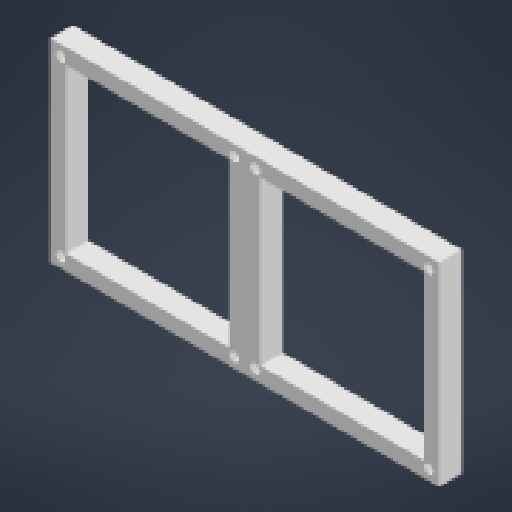
# Autodesk Inventor part: rack_2x1
Saved by Autodesk Inventor 2024 (Build 280153000, 153)
## iProperties
Created: 2026-04-07
Part Number: rack_2x1
Material: Generic
Document SubType Name: Modeling
Designer: schar
Density: 1 g/cm^3
Appearance: Default
Author: schar
Autodesk Inventor part; units mm, degrees
ref_plane "YZ Plane" through (0, 0, 0) normal (1, 0, 0) x (0, 1, 0)
ref_plane "XZ Plane" through (0, 0, 0) normal (0, 1, 0) x (-1, 0, 0)
ref_plane "XY Plane" through (0, 0, 0) normal (0, 0, 1) x (1, 0, 0)
sketch "Sketch1" plane through (0, 0, 0) normal (0, 0, 1) x (1, 0, 0)
  line L0 (19, -25) -> (-19, -25) projected
  line L1 (25, 19) -> (25, -19) projected
  line L2 (-19, 25) -> (19, 25) projected
  line L3 (-19, 25) -> (19, 25) projected
  line L4 (-19, 25) -> (19, 25) projected
  line L5 (-24, -7) -> (-24, 7) projected
  line L6 (-25, -25) -> (-25, 25) projected
  line L7 (25, 19) -> (25, -19) projected
  line L8 (-25, 25) -> (25, 25)
  line L9 (25, 25) -> (25, -25)
  line L10 (25, -25) -> (-25, -25)
  line L11 (-25, -25) -> (-25, 25)
  line L12 (-25.2, 25.2) -> (25.2, 25.2)
  line L13 (25.2, 25.2) -> (25.2, -25.2)
  line L14 (25.2, -25.2) -> (-25.2, -25.2)
  line L15 (-25.2, -25.2) -> (-25.2, 25.2)
  line L16 (-25.2, 25.2) -> (25.2, -25.2) construction
  line L17 (25.2, 25.2) -> (-25.2, -25.2) construction
  line L18 (-30, 30) -> (30, 30)
  line L19 (30, 30) -> (30, -30)
  line L20 (30, -30) -> (-30, -30)
  line L21 (-30, -30) -> (-30, 30)
  line L22 (-30, 30) -> (30, -30) construction
  line L23 (30, 30) -> (-30, -30) construction
  line L24 (-30, -30) -> (-30, 30)
  circle A0 centre (-26.7678, 26.7678) radius 1.5 projected
  circle A1 centre (-26.7678, 26.7678) radius 1.5
  circle A2 centre (26.7678, 26.7678) radius 1.5 projected
  circle A3 centre (26.7678, -26.7678) radius 1.5 projected
  circle A4 centre (-26.7678, -26.7678) radius 1.5 projected
  circle A5 centre (26.7678, 26.7678) radius 1.5
  circle A6 centre (26.7678, -26.7678) radius 1.5
  circle A7 centre (-26.7678, -26.7678) radius 1.5
  line L25 (-41, 25) -> (-79, 25)
  line L26 (-35, 25) -> (-85, 25)
  line L27 (-34.8, 25.2) -> (-85.2, 25.2)
  line L28 (-85.2, 25.2) -> (-85.2, -25.2)
  line L29 (-85.2, -25.2) -> (-34.8, -25.2)
  line L30 (-34.8, -25.2) -> (-34.8, 25.2)
  line L31 (-30, 30) -> (-90, 30)
  line L32 (-90, 30) -> (-90, -30)
  line L33 (-90, -30) -> (-30, -30)
  circle A8 centre (-33.2322, 26.7678) radius 1.5
  circle A9 centre (-33.2322, -26.7678) radius 1.5
  circle A10 centre (-86.7678, 26.7678) radius 1.5
  circle A11 centre (-86.7678, -26.7678) radius 1.5
  point P0 (0, 0)
  dimension "d0" = 50.4
  dimension "d1" = 50.4
  dimension "d2" = 60
  dimension "d3" = 60
  constraints: 52 end point, 15 symmetric about line, 8 centre point, 6 parallel, 5 coincident, 4 midpoint, 3 concentric, 3 horizontal, 3 perpendicular, 4 other
  measures "d0" distance of L13.end L14.end
  measures "d1" distance of L12.end L13.end
  measures "d2" distance of L19.end L20.end
  measures "d3" distance of L18.end L19.end
extrude "Extrusion1" add sketch "Sketch1" along normal blind 7 contours L18 L19 L20 L21 | L21 L33 L32 L31
body "Solid1"
